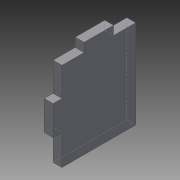
# Autodesk Inventor part: Back support
Saved by Autodesk Inventor 2015 (Build 190159000, 159)
## iProperties
Created: 2014-08-15
Part Number: Back support
Material: Generic
Document SubType Name: Modeling
Designer: karl
Density: 1 g/cm^3
Appearance: Default
Author: karl
Autodesk Inventor part; units mm, degrees
ref_plane "YZ Plane" through (0, 0, 0) normal (1, 0, 0) x (0, 1, 0)
ref_plane "XZ Plane" through (0, 0, 0) normal (0, 1, 0) x (-1, 0, 0)
ref_plane "XY Plane" through (0, 0, 0) normal (0, 0, 1) x (1, 0, 0)
sketch "Sketch1" plane through (0, 0, 0) normal (1, 0, 0) x (0, 1, 0)
  line L0 (-12.5, 10) -> (12.5, 10)
  line L1 (12.5, 10) -> (12.5, -10)
  line L2 (12.5, -10) -> (-12.5, -10)
  line L3 (-12.5, -10) -> (-12.5, 10)
  line L4 (-12.5, 10) -> (12.5, -10) construction
  line L5 (12.5, 10) -> (-12.5, -10) construction
  line L6 (5, 10) -> (-5, 10)
  line L7 (-5, 10) -> (-5, 13)
  line L8 (-5, 13) -> (5, 13)
  line L9 (5, 13) -> (5, 10)
  line L10 (-12.5, 5) -> (-15.5, 5)
  line L11 (-15.5, 5) -> (-15.5, -5)
  line L12 (-15.5, -5) -> (-12.5, -5)
  line L13 (-12.5, -5) -> (-12.5, 5)
  circle A0 centre (0, -10) radius 10
  point P0 (0, 0)
  point P1 (0, 13)
  point P2 (0, 0)
  dimension "d0" = 25
  dimension "d1" = 20
  dimension "d2" = 10
  dimension "d3" = 3
  dimension "d4" = 3
  dimension "d5" = 10
  dimension "d8" = 5
  constraints: 28 end point, 6 parallel, 5 midpoint, 3 horizontal, 3 perpendicular, 2 point on line, 2 vertical alignment, 2 other
  measures "d0" distance of L1.end L2.end
  measures "d1" distance of L0.end L1.end
  measures "d2" distance of L7.end L8.end
  measures "d3" distance of L6.end L7.end
  measures "d4" distance of L12.end L11.end
  measures "d5" distance of L11.end L10.end
  measures "d8" distance between parallel lines of L0 L10
extrude "Extrusion1" add sketch "Sketch1" along normal blind 3 contours L0 L1 L2 A0 L3 | L7 L8 L9 L0 | L3 L12 L11 L10 | A0 L2 picked at (-0.8971, -4.5365)
body "Solid1"
